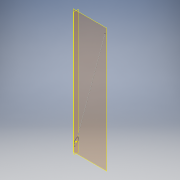
# Autodesk Inventor part: SingleUpperLine
Saved by Autodesk Inventor 2016 (Build 200138000, 138)
## iProperties
Created: 2016-01-20
Part Number: SingleUpperLine
Material: Generic
Document SubType Name: Modeling
Designer: KA ROSIE
Density: 1 g/cm^3
Appearance: Default
Author: KA ROSIE
Autodesk Inventor part; units mm, degrees
ref_plane "XZ Plane" through (0, 0, 0) normal (0, 1, 0) x (-1, 0, 0)
ref_plane "Work Plane1" through (0, 0, 0) normal (0.9659, -0.2588, 0) x (0, 0, 1)
ref_plane "Work Plane2" through (0, 0, 0) normal (0.2588, 0.9659, 0) x (0, 0, 1)
sketch "Sketch1" plane through (0, 0, 0) normal (0.9659, -0.2588, 0) x (0, 0, 1)
  ellipse E0 centre (0, 0) end of major axis (0, 75) minor radius 28.5189
  point P0 (28.5189, 0)
  dimension "d2" = 75
  constraints: 1 coincident, 1 horizontal alignment, 2 other
sketch "Sketch3" plane through (0, 0, 0) normal (0.2588, 0.9659, 0) x (0, 0, 1)
  point P0 (0, 0)
sketch "Sketch4" plane through (0, 0, 0) normal (0.2588, 0.9659, 0) x (0, 0, 1)
  line L0 (-14, 0) -> (14, 0) projected
  point P0 (0, 0)
sketch "Sketch5" plane through (0, 0, 0) normal (0.2588, 0.9659, 0) x (0, 0, 1)
  circle A0 centre (28.5391, 0) radius 3
  point P0 (0, 0)
  dimension "d3" = 6
  constraints: 1 centre point
  measures "d3" diameter of A0
sweep "Sweep1" add profiles "Sketch5" path "Sketch1"
sketch "Sketch6" plane through (0, 0, 0) normal (0.2588, 0.9659, 0) x (0, 0, 1)
  circle A0 centre (0, 0) radius 3
  dimension "d6" = 6
  constraints: 1 centre point, 1 coincident
  measures "d6" diameter of A0
extrude "Extrusion1" add sketch "Sketch6" along normal blind 1800
ref_plane "Work Plane3" through (16.5189, 73.2404, 0) normal (0.2588, 0.9659, 0) x (0, 0, 1)
sketch "Sketch7" plane through (0, 0, 0) normal (-0.2588, -0.9659, 0) x (0.9659, -0.2588, 0)
  circle A0 centre (0, 0) radius 3
  point P0 (0, 0)
  constraints: 1 centre point, 1 coincident
extrude "Extrusion2" cut sketch "Sketch7" against normal up to surface (75.0202 mm away)
body "Solid1"
